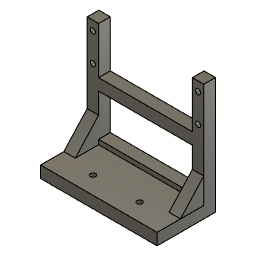
UselessBoxServoMountBiggerServo v1 (Autodesk Fusion 360 design; units mm, degrees)
Autodesk Fusion 360 part; units mm, degrees
note: some values were not read from the file. Set by a fixed rule: which sketch regions a step uses.
sketch "Sketch1" plane through (0, 0, 0) normal (0, 0, 1) x (1, 0, 0)
  line L0 (0, 0) -> (50, 0)
  line L1 (50, 0) -> (50, 50)
  line L2 (50, 50) -> (0, 50)
  line L3 (0, 50) -> (0, 0)
  line L4 (0, 50) -> (4.9, 50)
  line L5 (4.9, 50) -> (4.9, 29.9)
  line L6 (4.9, 29.9) -> (0, 29.9)
  line L7 (0, 29.9) -> (0, 50)
  line L8 (50, 50) -> (45.1, 50)
  line L9 (45.1, 50) -> (45.1, 29.9)
  line L10 (45.1, 29.9) -> (50, 29.9)
  line L11 (50, 29.9) -> (50, 50)
  line L12 (4.9, 29.9) -> (4.9, 24.9)
  line L13 (4.9, 24.9) -> (4.9, 0)
  line L14 (4.9, 0) -> (4.9, 7)
  line L15 (45.1, 29.9) -> (45.1, 0)
  line L16 (4.9, 24.9) -> (45.1, 24.9)
  line L17 (4.9, 7) -> (45.1, 7)
  line L18 (2.45, 50) -> (2.45, 29.9)
  line L19 (47.55, 50) -> (47.55, 29.9)
  line L20 (2.45, 29.9) -> (2.45, 33.9)
  line L21 (2.45, 50) -> (2.45, 46)
  line L22 (47.55, 50) -> (47.55, 46)
  line L23 (47.55, 29.9) -> (47.55, 33.9)
  circle A0 centre (2.45, 46) radius 1.1
  circle A1 centre (2.45, 33.9) radius 1.1
  circle A2 centre (47.55, 46) radius 1.1
  circle A3 centre (47.55, 33.9) radius 1.1
  line L24 (4.9, 29.9) -> (45.1, 29.9)
  dimension "d1" = 50
  dimension "d2" = 50
  dimension "d3" = 4.9
  dimension "d4" = 20.1
  dimension "d5" = 4.9
  dimension "d6" = 20.1
  dimension "d7" = 5
  dimension "d8" = 4
  dimension "d9" = 4
  dimension "d10" = 2.2
  dimension "d11" = 2.2
  dimension "d12" = 2.2
  dimension "d13" = 2.2
  constraint horizontal L0
  constraint vertical L1
  constraint horizontal L2
  constraint vertical L3
  constraint coincident L0.start L3.end
  constraint horizontal L4
  constraint vertical L5
  constraint horizontal L6
  constraint vertical L7
  constraint horizontal L8
  constraint vertical L9
  constraint horizontal L10
  constraint vertical L11
  constraint perpendicular L6 L12
  constraint coincident L0 L13.end
  constraint perpendicular L0 L13
  constraint coincident L13 L14.end
  constraint coincident L0 L15.end
  constraint perpendicular L0 L15
  constraint coincident L15 L16.end
  constraint perpendicular L15 L16
  constraint coincident L15 L17.end
  constraint perpendicular L15 L17
  constraint midpoint L4 L18.start
  constraint midpoint L6 L18.end
  constraint midpoint L8 L19.start
  constraint midpoint L10 L19.end
  constraint perpendicular L6 L20
  constraint coincident L18 L21.end
  constraint coincident L19 L22.end
  constraint perpendicular L8 L22
  constraint perpendicular L10 L23
  constraint coincident L21.end A0.centre
  constraint coincident L20.end A1.centre
  constraint coincident L22.end A2.centre
  constraint coincident L23.end A3.centre
  measures "d1" distance of L0.start L0.end
  measures "d2" distance of L0.start L2.end
  measures "d3" distance of L2.end L4.end
  measures "d4" distance of L2.end L6.end
  measures "d5" distance of L1.end L8.end
  measures "d6" distance of L1.end L10.end
  measures "d7" distance of L5.end L12.end
  measures "d8" distance of L18.end L20.end
  measures "d9" distance of L19.end L23.end
  measures "d10" diameter of A0
  measures "d11" diameter of A1
  measures "d12" diameter of A2
  measures "d13" diameter of A3
extrude "Extrude1" add sketch "Sketch1" along normal blind 5 contours L0 L3 L6 L12 L13 L14 | L0 L13 L14 L15 L17 | L2 L3 L4 L6 L7 L18 L20 L21 A0 A1 | L0 L1 L10 L15 | L2 L4 L5 L6 L18 L20 L21 A0 A1 | L12 L15 L16 L24 | L1 L2 L8 L10 L11 L19 L22 L23 A2 A3 | L2 L8 L9 L10 L19 L22 L23 A2 A3
sketch "Sketch2" plane through (0, 0, 5) normal (0, 0, 1) x (1, 0, 0)
  line L0 (4.9, 7) -> (4.9, 24.9)
  line L1 (4.9, 24.9) -> (45.1, 24.9)
  line L2 (45.1, 24.9) -> (45.1, 7)
  line L3 (45.1, 7) -> (4.9, 7)
  circle A0 centre (2.45, 33.9) radius 1.1
  circle A1 centre (47.55, 33.9) radius 1.1
  circle A2 centre (47.55, 46) radius 1.1
  circle A3 centre (2.45, 46) radius 1.1
  line L4 (0, 50) -> (0, 0)
  line L5 (0, 0) -> (50, 0)
  line L6 (50, 0) -> (50, 50)
  line L7 (50, 50) -> (45.1, 50)
  line L8 (45.1, 50) -> (45.1, 29.9)
  line L9 (45.1, 29.9) -> (4.9, 29.9)
  line L10 (4.9, 29.9) -> (4.9, 50)
  line L11 (4.9, 50) -> (0, 50)
  line L12 (0, 0) -> (50, 0)
  line L13 (50, 0) -> (50, 5)
  line L14 (50, 5) -> (0, 5)
  line L15 (0, 5) -> (0, 0)
  dimension "d16" = 5
  constraint horizontal L12
  constraint vertical L13
  constraint horizontal L14
  constraint vertical L15
  constraint coincident L4.end L5.start
  measures "d16" distance of L4.end L14.end
extrude "Extrude2" add sketch "Sketch2" along normal blind 20 contours L4 L5 L6 L12 L13 L14 L15
sketch "Sketch3" plane through (0, 0, 5) normal (0, 0, 1) x (1, 0, 0)
  line L0 (0, 5) -> (50, 5)
  line L1 (50, 5) -> (50, 50)
  line L2 (50, 50) -> (45.1, 50)
  line L3 (45.1, 50) -> (45.1, 29.9)
  line L4 (45.1, 29.9) -> (4.9, 29.9)
  line L5 (4.9, 29.9) -> (4.9, 50)
  line L6 (4.9, 50) -> (0, 50)
  line L7 (0, 50) -> (0, 5)
  line L8 (4.9, 7) -> (4.9, 24.9)
  line L9 (4.9, 24.9) -> (45.1, 24.9)
  line L10 (45.1, 24.9) -> (45.1, 7)
  line L11 (45.1, 7) -> (4.9, 7)
  circle A0 centre (2.45, 33.9) radius 1.1
  circle A1 centre (47.55, 33.9) radius 1.1
  circle A2 centre (47.55, 46) radius 1.1
  circle A3 centre (2.45, 46) radius 1.1
  line L12 (4.9, 5) -> (4.9, 15.95)
  line L13 (0, 15.95) -> (4.9, 15.95)
  line L14 (0, 15.95) -> (0, 5)
  line L15 (0, 5) -> (4.9, 5)
  line L16 (45.1, 15.95) -> (50, 15.95)
  line L17 (50, 15.95) -> (50, 5)
  line L18 (45.1, 15.95) -> (45.1, 5)
  constraint coincident L0 L12.start
  constraint midpoint L8 L12.end
  constraint perpendicular L11 L12
  constraint coincident L7 L13.start
  constraint perpendicular L8 L13
  constraint coincident L0.start L7.end
  constraint midpoint L10 L16.start
  constraint coincident L1 L16.end
  constraint perpendicular L1 L16
  constraint coincident L0.end L1.start
  constraint coincident L0 L18.end
  constraint perpendicular L0 L18
extrude "Extrude3" add sketch "Sketch3" along normal blind 10 contours L0 L7 L8 L12 L13 L14 L15 | L0 L1 L10 L16 L17 L18
sketch "Sketch4" plane through (0, 0, 0) normal (-1, 0, 0) x (0, 0, 1)
  line L0 (0, 50) -> (0, 0)
  line L1 (0, 0) -> (25, 0)
  line L2 (25, 0) -> (25, 5)
  line L3 (25, 5) -> (15, 5)
  line L4 (15, 5) -> (15, 15.95)
  line L5 (15, 15.95) -> (5, 15.95)
  line L6 (5, 15.95) -> (5, 50)
  line L7 (5, 50) -> (0, 50)
  line L8 (5, 15.95) -> (15, 5)
  constraint coincident L5.end L6.start
  constraint coincident L3.end L4.start
extrude "Extrude4" cut sketch "Sketch4" against normal blind 5 contours L4 L5 L8
sketch "Sketch5" plane through (50, 0, 0) normal (1, 0, 0) x (0, 0, -1)
  line L0 (-5, 5) -> (-5, 15.95)
  line L1 (-5, 15.95) -> (-15, 15.95)
  line L2 (-15, 15.95) -> (-15, 5)
  line L3 (-15, 5) -> (-5, 5)
  line L4 (-5, 15.95) -> (-15, 5)
  constraint coincident L0.end L1.start
  constraint coincident L2.end L3.start
extrude "Extrude5" cut sketch "Sketch5" against normal blind 5 contours L1 L2 L4
sketch "Sketch6" plane through (0, 5, 0) normal (0, 1, 0) x (-1, 0, 0)
  line L0 (-4.9, 5) -> (-4.9, 15)
  line L1 (-4.9, 15) -> (0, 15)
  line L2 (0, 15) -> (0, 25)
  line L3 (0, 25) -> (-50, 25)
  line L4 (-50, 25) -> (-50, 15)
  line L5 (-50, 15) -> (-45.1, 15)
  line L6 (-45.1, 15) -> (-45.1, 5)
  line L7 (-45.1, 5) -> (-4.9, 5)
  line L8 (0, 25) -> (-15, 25)
  line L9 (-15, 25) -> (-15, 17.5)
  line L10 (-15, 17.5) -> (0, 17.5)
  line L11 (0, 17.5) -> (0, 25)
  line L12 (-50, 25) -> (-35, 25)
  line L13 (-35, 25) -> (-35, 17.5)
  line L14 (-35, 17.5) -> (-50, 17.5)
  line L15 (-50, 17.5) -> (-50, 25)
  circle A0 centre (-15, 17.5) radius 1.125
  circle A1 centre (-35, 17.5) radius 1.125
  dimension "d25" = 15
  dimension "d26" = 7.5
  dimension "d27" = 15
  dimension "d28" = 7.5
  dimension "d29" = 2.25
  dimension "d30" = 2.25
  constraint horizontal L8
  constraint vertical L9
  constraint horizontal L10
  constraint vertical L11
  constraint coincident L2.end L3.start
  constraint horizontal L12
  constraint vertical L13
  constraint horizontal L14
  constraint vertical L15
  constraint coincident L3.end L4.start
  constraint coincident L9.end L10.start
  constraint coincident L13.end L14.start
  measures "d25" distance of L2.end L8.end
  measures "d26" distance of L2.end L10.end
  measures "d27" distance of L3.end L12.end
  measures "d28" distance of L3.end L14.end
  measures "d29" diameter of A0
  measures "d30" diameter of A1
extrude "Extrude6" cut sketch "Sketch6" against normal blind 5 contours L9 L10 A0 | L9 L10 A0 | L13 L14 A1 | L13 L14 A1
